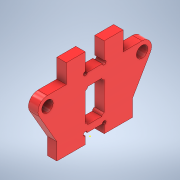
# Autodesk Inventor part: hw8
Saved by Autodesk Inventor 2021 (Build 250183000, 183)
## iProperties
Created: 2022-04-30
Part Number: hw8
Material: Generic
Document SubType Name: Modeling
Designer: authe
Density: 1 g/cm^3
Appearance: Light Red
Author: authe
Autodesk Inventor part; units mm, degrees
ref_plane "YZ Plane" through (0, 0, 0) normal (1, 0, 0) x (0, 1, 0)
ref_plane "XZ Plane" through (0, 0, 0) normal (0, 1, 0) x (-1, 0, 0)
ref_plane "XY Plane" through (0, 0, 0) normal (0, 0, 1) x (1, 0, 0)
sketch "Sketch1" plane through (0, 0, 0) normal (1, 0, 0) x (0, 1, 0)
  line L0 (8, 10) -> (0, 10)
  line L1 (0, 10) -> (0, 40)
  line L2 (0, 40) -> (17.6795, 40)
  arc A0 (65, 50) -> (50, 58.6603) centre (55, 50) ccw
  line L3 (65, 50) -> (65, 40)
  line L4 (61.5, 0) -> (66, 0)
  line L5 (65, 40) -> (65, 30)
  line L6 (65, 30) -> (85, 30)
  line L7 (85, 30) -> (85, 10)
  line L8 (10, 8) -> (10, 0)
  line L9 (50, 58.6603) -> (17.6795, 40)
  circle A1 centre (55, 50) radius 6
  line L10 (85, 10) -> (67, 10)
  line L11 (65, 8) -> (65, 0)
  line L12 (49.5, 10) -> (19.5, 10)
  line L13 (17, 7.5) -> (17, 0)
  line L14 (17, 0) -> (52, 0)
  line L15 (52, 0) -> (52, 7.5)
  arc A2 (67, 10) -> (65, 8) centre (65, 10) ccw
  arc A3 (49.5, 10) -> (52, 7.5) centre (52, 10) ccw
  arc A4 (17, 7.5) -> (19.5, 10) centre (17, 10) ccw
  arc A5 (10, 8) -> (8, 10) centre (10, 10) ccw
  line L16 (65, -40) -> (65, -30)
  arc A6 (52, -7.5) -> (49.5, -10) centre (52, -10) ccw
  line L17 (52, 0) -> (52, -7.5)
  line L18 (65, -50) -> (65, -40)
  arc A7 (50, -58.6603) -> (65, -50) centre (55, -50) ccw
  line L19 (49.5, -10) -> (19.5, -10)
  line L20 (50, -58.6603) -> (17.6795, -40)
  arc A8 (19.5, -10) -> (17, -7.5) centre (17, -10) ccw
  circle A9 centre (55, -50) radius 6
  line L21 (8, -10) -> (0, -10)
  line L22 (0, -10) -> (0, -40)
  line L23 (0, -40) -> (17.6795, -40)
  line L24 (17, -7.5) -> (17, 0)
  arc A10 (8, -10) -> (10, -8) centre (10, -10) ccw
  line L25 (10, -8) -> (10, 0)
  line L26 (65, -30) -> (85, -30)
  line L27 (85, -30) -> (85, -10)
  line L28 (65, -8) -> (65, 0)
  arc A11 (65, -8) -> (67, -10) centre (65, -10) ccw
  line L29 (85, -10) -> (67, -10)
  line L30 (17.6795, 40) -> (28.4601, 40)
  point P0 (0, 0)
  point P1 (0, 0)
  dimension "d21" = 35
  dimension "d22" = 55
  dimension "d23" = 85
  dimension "d24" = 12
  dimension "d25" = 2.5
  dimension "d26" = 20
  dimension "d27" = 80
  dimension "d28" = 20
  dimension "d29" = 100
  dimension "d32" = 30
  constraints: 62 end point, 26 symmetric about line, 20 point on circle, 12 centre point, 8 coincident, 5 perpendicular, 4 horizontal, 3 parallel, 2 tangent, 2 vertical, 1 point on line, 6 other
  measures "d21" distance of L24.end L17.start
  measures "d22" distance of L8.end L11.end
  measures "d23" distance of L21.end L29.start
  measures "d24" diameter of A9
  measures "d25" distance of L19.start A6.centre
  measures "d26" distance of L26.end L29.start
  measures "d27" distance of L23.start L1.end
  measures "d28" distance of L21.end L0.end
  measures "d29" distance of A7.centre A0.centre
  measures "d32" angle of L9 L30
sketch "Sketch2" plane through (0, 0, 0) normal (1, 0, 0) x (0, 1, 0)
  point P0 (0, 0)
extrude "Extrusion1" add sketch "Sketch1" along normal mid plane 10
body "Solid1"
